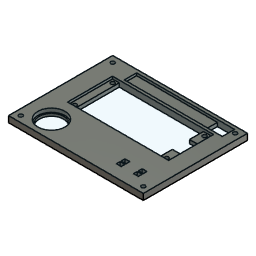
Arduino_MountingPlate_v4 (Autodesk Fusion 360 design; units mm, degrees)
Autodesk Fusion 360 part; units mm, degrees
sketch "Sketch1" plane through (0, 0, 0) normal (0, 1, 0) x (1, 0, 0) in component "mountingPlatee"
  line L0 (0, 0) -> (110, 0)
  line L1 (110, 0) -> (110, -85)
  line L2 (110, -85) -> (0, -85)
  line L3 (0, -85) -> (0, 0)
  line L4 (15, -15) -> (95, -15)
  line L5 (95, -15) -> (95, -51)
  line L6 (95, -51) -> (15, -51)
  line L7 (15, -51) -> (15, -15)
  line L8 (15, -15) -> (15, -17.5)
  circle A0 centre (17.5, -17.5) radius 1.6
  line L9 (15, -51) -> (17.5, -51)
  line L10 (15, -48.5) -> (15, -51)
  circle A1 centre (17.5, -48.5) radius 1.6
  circle A2 centre (92.5, -48.5) radius 1.6
  circle A3 centre (92.5, -17.5) radius 1.6
  line L11 (15, -15) -> (20, -15)
  line L12 (20, -15) -> (20, -51)
  line L13 (20, -51) -> (15, -51)
  line L14 (15, -51) -> (15, -15)
  line L15 (95, -15) -> (88.7416, -15)
  line L16 (88.7416, -15) -> (88.7416, -51)
  line L17 (88.7416, -51) -> (95, -51)
  line L18 (95, -51) -> (95, -15)
  line L19 (22, -2.5) -> (88, -2.5)
  line L20 (88, -2.5) -> (88, -12.5)
  line L21 (88, -12.5) -> (22, -12.5)
  line L22 (22, -12.5) -> (22, -2.5)
  circle A4 centre (20, -70) radius 10
  circle A5 centre (5, -80) radius 1.6
  circle A6 centre (5, -5) radius 1.6
  circle A7 centre (105, -5) radius 1.6
  circle A8 centre (105, -80) radius 1.6
  line L23 (95, -68) -> (92, -68)
  line L24 (95, -75) -> (92, -75)
  line L25 (92, -71) -> (95, -71)
  line L26 (95, -72) -> (92, -72)
  line L27 (82, -68) -> (79, -68)
  line L28 (79, -71) -> (82, -71)
  line L29 (82, -71) -> (82, -68)
  line L30 (82, -72) -> (79, -72)
  line L31 (79, -75) -> (82, -75)
  line L32 (82, -75) -> (82, -72)
  line L33 (88, -2.5) -> (102, -2.5)
  line L34 (102, -2.5) -> (102, -12.5)
  line L35 (102, -12.5) -> (88, -12.5)
  line L36 (88, -12.5) -> (88, -2.5)
  circle A9 centre (20, -70) radius 11.1
  line L37 (92, -75) -> (96, -75)
  line L38 (96, -75) -> (96, -72)
  line L39 (96, -72) -> (92, -72)
  line L40 (92, -72) -> (92, -75)
  line L41 (92, -71) -> (96, -71)
  line L42 (96, -71) -> (96, -68)
  line L43 (96, -68) -> (92, -68)
  line L44 (92, -68) -> (92, -71)
  line L45 (82, -75) -> (78, -75)
  line L46 (78, -75) -> (78, -72)
  line L47 (78, -72) -> (82, -72)
  line L48 (82, -72) -> (82, -75)
  line L49 (82, -71) -> (78, -71)
  line L50 (78, -71) -> (78, -68)
  line L51 (78, -68) -> (82, -68)
  line L52 (82, -68) -> (82, -71)
  dimension "d3" = 110
  dimension "d4" = 85
  dimension "d5" = 80
  dimension "d6" = 36
  dimension "d9" = 3.2
  dimension "d12" = 3.2
  dimension "d15" = 3.2
  dimension "d16" = 3.2
  dimension "d24" = 3.2
  dimension "d25" = 3.2
  dimension "d26" = 3.2
  dimension "d27" = 3.2
  dimension "d30" = 14
  dimension "d31" = 10
  dimension "d32" = 22.2
  constraint horizontal L0
  constraint vertical L1
  constraint horizontal L2
  constraint vertical L3
  constraint horizontal L4
  constraint vertical L5
  constraint horizontal L6
  constraint vertical L7
  constraint coincident L7 L8.end
  constraint horizontal L11
  constraint vertical L12
  constraint horizontal L13
  constraint vertical L14
  constraint coincident L6 L12.end
  constraint horizontal L15
  constraint vertical L16
  constraint horizontal L17
  constraint vertical L18
  constraint coincident L6 L16.end
  constraint horizontal L19
  constraint vertical L20
  constraint horizontal L21
  constraint vertical L22
  constraint horizontal L23
  constraint horizontal L24
  constraint horizontal L25
  constraint horizontal L26
  constraint horizontal L27
  constraint horizontal L28
  constraint vertical L29
  constraint horizontal L30
  constraint horizontal L31
  constraint vertical L32
  constraint horizontal L33
  constraint vertical L34
  constraint horizontal L35
  constraint vertical L36
  constraint concentric A4 A9
  constraint horizontal L37
  constraint vertical L38
  constraint horizontal L39
  constraint vertical L40
  constraint horizontal L41
  constraint vertical L42
  constraint horizontal L43
  constraint vertical L44
  constraint horizontal L45
  constraint vertical L46
  constraint horizontal L47
  constraint vertical L48
  constraint horizontal L49
  constraint vertical L50
  constraint horizontal L51
  constraint vertical L52
  measures "d3" distance of L0.start L0.end
  measures "d4" distance of L0.start L2.end
  measures "d5" distance of L4.start L4.end
  measures "d6" distance of L4.start L6.end
  measures "d9" diameter of A0
  measures "d12" diameter of A1
  measures "d15" diameter of A2
  measures "d16" diameter of A3
  measures "d24" diameter of A5
  measures "d25" diameter of A6
  measures "d26" diameter of A7
  measures "d27" diameter of A8
  measures "d30" distance of L19.end L33.end
  measures "d31" distance of L19.end L20.end
  measures "d32" diameter of A9
sketch "Sketch1 (2)" plane through (0, 0, 0) normal (0, 1, 0) x (1, 0, 0)
sketch "Sketch2" plane through (0, 0, 0) normal (0, 1, 0) x (1, 0, 0)
extrude "Extrude1" add sketch "Sketch1" along normal blind 5 contours L0 L1 L2 L3 | L4 L6 L7 L8 L9 L10 L11 L12 L13 L14 | L4 L5 L6 L15 L16 L17 L18 | L19 L20 L21 L22 L36 | A9
sketch "Sketch3" plane through (0, 5, 0) normal (0, 1, 0) x (-1, 0, 0)
  line L0 (-92, 75) -> (-92, 72)
  line L1 (-92, 72) -> (-96, 72)
  line L2 (-96, 72) -> (-96, 75)
  line L3 (-96, 75) -> (-92, 75)
  circle A0 centre (-5, 5) radius 1.6
  circle A1 centre (-17.5, 17.5) radius 1.6
  line L4 (-102, 12.5) -> (-88, 12.5)
  line L5 (-88, 12.5) -> (-88, 2.5)
  line L6 (-88, 2.5) -> (-102, 2.5)
  line L7 (-102, 2.5) -> (-102, 12.5)
  circle A2 centre (-105, 5) radius 1.6
  circle A3 centre (-105, 80) radius 1.6
  circle A4 centre (-17.5, 48.5) radius 1.6
  line L8 (-92, 71) -> (-92, 68)
  line L9 (-92, 68) -> (-96, 68)
  line L10 (-96, 68) -> (-96, 71)
  line L11 (-96, 71) -> (-92, 71)
  circle A5 centre (-5, 80) radius 1.6
  line L12 (-78, 68) -> (-82, 68)
  line L13 (-82, 68) -> (-82, 71)
  line L14 (-82, 71) -> (-78, 71)
  line L15 (-78, 71) -> (-78, 68)
  circle A6 centre (-92.5, 17.5) radius 1.6
  line L16 (-78, 72) -> (-82, 72)
  line L17 (-82, 72) -> (-82, 75)
  line L18 (-82, 75) -> (-78, 75)
  line L19 (-78, 75) -> (-78, 72)
  line L20 (-20, 51) -> (-20, 15)
  line L21 (-20, 15) -> (-88.7416, 15)
  line L22 (-88.7416, 15) -> (-88.7416, 51)
  line L23 (-88.7416, 51) -> (-20, 51)
  circle A7 centre (-92.5, 48.5) radius 1.6
  circle A8 centre (-20, 70) radius 10
  line L24 (0, 85) -> (-110, 85)
  line L25 (-110, 85) -> (-110, 0)
  line L26 (-110, 0) -> (0, 0)
  line L27 (0, 0) -> (0, 85)
  line L28 (-88, 2.5) -> (-22, 2.5)
  line L29 (-22, 2.5) -> (-22, 12.5)
  line L30 (-22, 12.5) -> (-88, 12.5)
  line L31 (-88, 12.5) -> (-88, 2.5)
  circle A9 centre (-20, 70) radius 11.1
  dimension "d35" = 66
  dimension "d36" = 22.2
  constraint horizontal L28
  constraint vertical L29
  constraint horizontal L30
  constraint vertical L31
  constraint coincident L5.end L6.start
  constraint concentric A8 A9
  measures "d35" distance of L5.end L28.end
  measures "d36" diameter of A9
extrude "Extrude2" cut sketch "Sketch3" against normal blind 2 contours L5 L28 L29 L30 L31 | A9
extrude "Extrude3" cut 1 faces at (30.692, 3, 70.5515) along direction (0, -1, 0) blind 1
sketch "Sketch4" plane through (0, 5, 0) normal (0, 1, 0) x (-1, 0, 0)
  line L0 (-22, 2.5) -> (-102, 2.5)
  line L1 (-102, 2.5) -> (-102, 12.5)
  line L2 (-102, 12.5) -> (-22, 12.5)
  line L3 (-22, 12.5) -> (-22, 2.5)
  circle A0 centre (-20, 70) radius 11.1
  line L4 (-92, 75) -> (-92, 72)
  line L5 (-92, 72) -> (-96, 72)
  line L6 (-96, 72) -> (-96, 75)
  line L7 (-96, 75) -> (-92, 75)
  circle A1 centre (-5, 5) radius 1.6
  circle A2 centre (-17.5, 17.5) radius 1.6
  circle A3 centre (-105, 5) radius 1.6
  circle A4 centre (-105, 80) radius 1.6
  circle A5 centre (-17.5, 48.5) radius 1.6
  line L8 (-92, 71) -> (-92, 68)
  line L9 (-92, 68) -> (-96, 68)
  line L10 (-96, 68) -> (-96, 71)
  line L11 (-96, 71) -> (-92, 71)
  circle A6 centre (-5, 80) radius 1.6
  line L12 (-78, 68) -> (-82, 68)
  line L13 (-82, 68) -> (-82, 71)
  line L14 (-82, 71) -> (-78, 71)
  line L15 (-78, 71) -> (-78, 68)
  circle A7 centre (-92.5, 17.5) radius 1.6
  line L16 (-78, 72) -> (-82, 72)
  line L17 (-82, 72) -> (-82, 75)
  line L18 (-82, 75) -> (-78, 75)
  line L19 (-78, 75) -> (-78, 72)
  line L20 (-20, 51) -> (-20, 15)
  line L21 (-20, 15) -> (-88.7416, 15)
  line L22 (-88.7416, 15) -> (-88.7416, 51)
  line L23 (-88.7416, 51) -> (-20, 51)
  circle A8 centre (-92.5, 48.5) radius 1.6
  line L24 (0, 85) -> (-110, 85)
  line L25 (-110, 85) -> (-110, 0)
  line L26 (-110, 0) -> (0, 0)
  line L27 (0, 0) -> (0, 85)
  line L28 (-20, 15) -> (-15, 15)
  line L29 (-15, 15) -> (-15, 51)
  line L30 (-15, 51) -> (-20, 51)
  line L31 (-20, 51) -> (-20, 15)
  line L32 (-88.7416, 15) -> (-96, 15)
  line L33 (-96, 15) -> (-96, 51)
  line L34 (-96, 51) -> (-88.7416, 51)
  line L35 (-88.7416, 51) -> (-88.7416, 15)
  line L36 (-88.7416, 51) -> (-88.7416, 40)
  line L37 (-88.7416, 40) -> (-96, 40)
  line L38 (-96, 40) -> (-96, 26)
  line L39 (-96, 26) -> (-88.7416, 26)
  line L40 (-88.7416, 26) -> (-88.7416, 40)
  constraint horizontal L28
  constraint vertical L29
  constraint horizontal L30
  constraint vertical L31
  constraint coincident L20.end L21.start
  constraint horizontal L32
  constraint vertical L33
  constraint horizontal L34
  constraint vertical L35
  constraint coincident L21.end L22.start
  constraint coincident L22 L36.end
  constraint perpendicular L21 L36
  constraint horizontal L37
  constraint vertical L38
  constraint horizontal L39
  constraint vertical L40
  constraint coincident L33 L38.end
extrude "Extrude4" cut sketch "Sketch4" against normal blind 5 contours L22 L33 L35 L37 L38 L39 L40
sketch "Sketch5" plane through (0, 5, 0) normal (0, 1, 0) x (-1, 0, 0)
  line L0 (-96, 40) -> (-88.7416, 40)
  line L1 (-88.7416, 40) -> (-88.7416, 51)
  line L2 (-88.7416, 51) -> (-20, 51)
  line L3 (-20, 51) -> (-20, 15)
  line L4 (-20, 15) -> (-88.7416, 15)
  line L5 (-88.7416, 15) -> (-88.7416, 26)
  line L6 (-88.7416, 26) -> (-96, 26)
  line L7 (-96, 26) -> (-96, 40)
  line L8 (-22, 2.5) -> (-102, 2.5)
  line L9 (-102, 2.5) -> (-102, 12.5)
  line L10 (-102, 12.5) -> (-22, 12.5)
  line L11 (-22, 12.5) -> (-22, 2.5)
  circle A0 centre (-20, 70) radius 11.1
  line L12 (-92, 75) -> (-92, 72)
  line L13 (-92, 72) -> (-96, 72)
  line L14 (-96, 72) -> (-96, 75)
  line L15 (-96, 75) -> (-92, 75)
  circle A1 centre (-5, 5) radius 1.6
  circle A2 centre (-17.5, 17.5) radius 1.6
  circle A3 centre (-105, 5) radius 1.6
  circle A4 centre (-105, 80) radius 1.6
  circle A5 centre (-17.5, 48.5) radius 1.6
  line L16 (-92, 71) -> (-92, 68)
  line L17 (-92, 68) -> (-96, 68)
  line L18 (-96, 68) -> (-96, 71)
  line L19 (-96, 71) -> (-92, 71)
  circle A6 centre (-5, 80) radius 1.6
  line L20 (-78, 68) -> (-82, 68)
  line L21 (-82, 68) -> (-82, 71)
  line L22 (-82, 71) -> (-78, 71)
  line L23 (-78, 71) -> (-78, 68)
  circle A7 centre (-92.5, 17.5) radius 1.6
  line L24 (-78, 72) -> (-82, 72)
  line L25 (-82, 72) -> (-82, 75)
  line L26 (-82, 75) -> (-78, 75)
  line L27 (-78, 75) -> (-78, 72)
  circle A8 centre (-92.5, 48.5) radius 1.6
  line L28 (0, 85) -> (-110, 85)
  line L29 (-110, 85) -> (-110, 0)
  line L30 (-110, 0) -> (0, 0)
  line L31 (0, 0) -> (0, 85)
  line L32 (-20, 15) -> (-14.5, 15)
  line L33 (-14.5, 15) -> (-14.5, 51)
  line L34 (-14.5, 51) -> (-20, 51)
  line L35 (-20, 51) -> (-20, 15)
  line L36 (-88.7416, 15) -> (-97, 15)
  line L37 (-97, 15) -> (-97, 26)
  line L38 (-97, 26) -> (-88.7416, 26)
  line L39 (-88.7416, 26) -> (-88.7416, 15)
  line L40 (-88.7416, 40) -> (-97, 40)
  line L41 (-97, 40) -> (-97, 51)
  line L42 (-97, 51) -> (-88.7416, 51)
  line L43 (-88.7416, 51) -> (-88.7416, 40)
  dimension "d43" = 5.5
  dimension "d44" = 36
  constraint horizontal L32
  constraint vertical L33
  constraint horizontal L34
  constraint vertical L35
  constraint coincident L3.end L4.start
  constraint horizontal L36
  constraint vertical L37
  constraint horizontal L38
  constraint vertical L39
  constraint coincident L4.end L5.start
  constraint horizontal L40
  constraint vertical L41
  constraint horizontal L42
  constraint vertical L43
  constraint coincident L0.end L1.start
  measures "d43" distance of L3.end L32.end
  measures "d44" distance of L3.end L2.end
extrude "Extrude5" cut sketch "Sketch5" against normal blind 2 contours L0 L1 L40 L41 L42 L43 | L5 L6 L36 L37 L38 L39 | L3 L32 L33 L34 L35
sketch "Sketch6" plane through (0, 5, 0) normal (0, 1, 0) x (-1, 0, 0)
  line L0 (-14.5, 15) -> (-97, 15)
  line L1 (-97, 15) -> (-97, 26)
  line L2 (-97, 26) -> (-96, 26)
  line L3 (-96, 26) -> (-96, 40)
  line L4 (-96, 40) -> (-97, 40)
  line L5 (-97, 40) -> (-97, 51)
  line L6 (-97, 51) -> (-20, 51)
  line L7 (-20, 51) -> (-14.5, 51)
  line L8 (-14.5, 51) -> (-14.5, 15)
  line L9 (-22, 2.5) -> (-102, 2.5)
  line L10 (-102, 2.5) -> (-102, 12.5)
  line L11 (-102, 12.5) -> (-22, 12.5)
  line L12 (-22, 12.5) -> (-22, 2.5)
  circle A0 centre (-20, 70) radius 11.1
  line L13 (-92, 75) -> (-92, 72)
  line L14 (-92, 72) -> (-96, 72)
  line L15 (-96, 72) -> (-96, 75)
  line L16 (-96, 75) -> (-92, 75)
  circle A1 centre (-5, 5) radius 1.6
  circle A2 centre (-105, 5) radius 1.6
  circle A3 centre (-105, 80) radius 1.6
  line L17 (-92, 71) -> (-92, 68)
  line L18 (-92, 68) -> (-96, 68)
  line L19 (-96, 68) -> (-96, 71)
  line L20 (-96, 71) -> (-92, 71)
  circle A4 centre (-5, 80) radius 1.6
  line L21 (-78, 68) -> (-82, 68)
  line L22 (-82, 68) -> (-82, 71)
  line L23 (-82, 71) -> (-78, 71)
  line L24 (-78, 71) -> (-78, 68)
  line L25 (-78, 72) -> (-82, 72)
  line L26 (-82, 72) -> (-82, 75)
  line L27 (-82, 75) -> (-78, 75)
  line L28 (-78, 75) -> (-78, 72)
  line L29 (0, 85) -> (-110, 85)
  line L30 (-110, 85) -> (-110, 0)
  line L31 (-110, 0) -> (0, 0)
  line L32 (0, 0) -> (0, 85)
  line L33 (-97, 26) -> (-96, 26)
  line L34 (-96, 26) -> (-96, 40)
  line L35 (-96, 40) -> (-97, 40)
  line L36 (-97, 40) -> (-97, 26)
  constraint horizontal L33
  constraint vertical L34
  constraint horizontal L35
  constraint vertical L36
  constraint coincident L3.end L4.start
  constraint coincident L1.end L2.start
extrude "Extrude6" cut sketch "Sketch6" against normal blind 5 contours L2 L3 L4 L33 L34 L35 L36
extrude "Extrude7" cut 2 faces at (42.9139, 1, 51) (94.2472, 3.6667, 51) along direction (0, 0, 1) blind 0.3
extrude "Extrude8" cut 1 faces at (42.9139, 1, 15) along direction (0, 0, -1) blind 0.3
sketch "Sketch7" plane through (0, 5, 0) normal (0, 1, 0) x (-1, 0, 0)
  line L0 (-97, 14.7) -> (-97, 51.3)
  line L1 (-97, 51.3) -> (-20, 51.3)
  line L2 (-20, 51.3) -> (-14.5, 51.3)
  line L3 (-14.5, 51.3) -> (-14.5, 14.7)
  line L4 (-14.5, 14.7) -> (-97, 14.7)
  line L5 (0, 85) -> (-110, 85)
  line L6 (-110, 85) -> (-110, 0)
  line L7 (-110, 0) -> (0, 0)
  line L8 (0, 0) -> (0, 85)
  line L9 (-78, 72) -> (-82, 72)
  line L10 (-82, 72) -> (-82, 75)
  line L11 (-82, 75) -> (-78, 75)
  line L12 (-78, 75) -> (-78, 72)
  line L13 (-78, 68) -> (-82, 68)
  line L14 (-82, 68) -> (-82, 71)
  line L15 (-82, 71) -> (-78, 71)
  line L16 (-78, 71) -> (-78, 68)
  circle A0 centre (-5, 80) radius 1.6
  line L17 (-92, 71) -> (-92, 68)
  line L18 (-92, 68) -> (-96, 68)
  line L19 (-96, 68) -> (-96, 71)
  line L20 (-96, 71) -> (-92, 71)
  circle A1 centre (-105, 80) radius 1.6
  circle A2 centre (-105, 5) radius 1.6
  circle A3 centre (-5, 5) radius 1.6
  line L21 (-92, 75) -> (-92, 72)
  line L22 (-92, 72) -> (-96, 72)
  line L23 (-96, 72) -> (-96, 75)
  line L24 (-96, 75) -> (-92, 75)
  circle A4 centre (-20, 70) radius 11.1
  line L25 (-22, 2.5) -> (-102, 2.5)
  line L26 (-102, 2.5) -> (-102, 12.5)
  line L27 (-102, 12.5) -> (-22, 12.5)
  line L28 (-22, 12.5) -> (-22, 2.5)
component "mountingPlatee" placed x (1, 0, 0) y (0, 1, 0) z (0, 0, 1) at (0, 0, 0)
